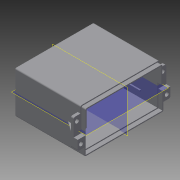
# Autodesk Inventor part: sensor2_2t
Saved by Autodesk Inventor 2015 (Build 190159000, 159)
## iProperties
Created: 2015-12-14
Part Number: sensor2_2t
Material: Generic
Document SubType Name: Modeling
Designer: mca20
Density: 1 g/cm^3
Appearance: Default
Author: mca20
Autodesk Inventor part; units mm, degrees
ref_plane "YZ Plane" through (0, 0, 0) normal (1, 0, 0) x (0, 1, 0)
ref_plane "XZ Plane" through (0, 0, 0) normal (0, 1, 0) x (-1, 0, 0)
ref_plane "XY Plane" through (0, 0, 0) normal (0, 0, 1) x (1, 0, 0)
sketch "Sketch1" plane through (0, 0, 0) normal (0, 1, 0) x (-1, 0, 0)
  line L0 (0, 0) -> (-48.5, 0)
  line L1 (-48.5, 0) -> (-48.5, -55)
  line L2 (-48.5, -55) -> (0, -55)
  line L3 (0, -55) -> (0, 0)
  line L4 (1.5, 1.5) -> (-50, 1.5)
  line L5 (-50, 1.5) -> (-50, -56.5)
  line L6 (-50, -56.5) -> (1.5, -56.5)
  line L7 (1.5, -56.5) -> (1.5, 1.5)
  dimension "d0" = 55
  dimension "d1" = 48.5
  dimension "d2" = 51.5
  dimension "d3" = 58
  dimension "d4" = 1.5
  dimension "d5" = 1.5
  constraints: 16 end point, 4 parallel, 2 horizontal, 2 perpendicular
  measures "d0" distance between parallel lines of L2 L0
  measures "d1" distance between parallel lines of L1 L3
  measures "d2" distance between parallel lines of L5 L7
  measures "d3" distance between parallel lines of L6 L4
  measures "d4" distance between parallel lines of L5 L1
  measures "d5" distance between parallel lines of L6 L2
extrude "Extrusion1" add sketch "Sketch1" against normal blind 1.5 contours L3 L2 L1 L0 | L7 L6 L5 L4
sketch "Sketch2" plane through (0, 0, 0) normal (0, 1, 0) x (1, 0, 0)
  line L0 (-1.5, -1.5) -> (50, -1.5)
  line L1 (50, 56.5) -> (-1.5, 56.5)
  line L2 (-1.5, 56.5) -> (-1.5, -1.5)
  line L3 (0, 0) -> (50, 0)
  line L4 (50, 55) -> (0, 55)
  line L5 (0, 55) -> (0, 0)
  line L6 (50, 0) -> (50, -1.5)
  line L7 (50, 56.5) -> (50, -1.5) projected
  line L8 (50, 55) -> (50, 56.5)
  line L9 (-1.5, 56.5) -> (50, 56.5) projected
  dimension "d8" = 55
  constraints: 16 end point, 2 horizontal, 2 parallel, 1 collinear, 1 perpendicular
  measures "d8" distance between parallel lines of L4 L3
extrude "Extrusion2" add sketch "Sketch2" along normal blind 28 contours L2 L1 L7 L4 L5 L3 L6 L0
sketch "Sketch3" plane through (0, 28, 0) normal (0, 1, 0) x (1, 0, 0)
  line L0 (-1.5, 56.5) -> (50, 56.5)
  line L1 (50, 56.5) -> (50, -1.5)
  line L2 (50, -1.5) -> (-1.5, -1.5)
  line L3 (-1.5, -1.5) -> (-1.5, 56.5)
  point P0 (0, 0)
  constraints: 8 end point, 2 parallel, 1 horizontal, 1 perpendicular
extrude "Extrusion3" add sketch "Sketch3" along normal blind 1.5
fillet "Fillet1" radius 1 8 edges at (24.25, 29.5, 1.5) (24.25, 29.5, -56.5) (-1.5, 29.5, -27.5) (-1.5, 14, 1.5) (24.25, -1.5, 1.5) (-1.5, -1.5, -27.5) (24.25, -1.5, -56.5) (-1.5, 14, -56.5)
sketch "Sketch4" plane through (0, 0, 0) normal (1, 0, 0) x (0, 0, -1)
  line L0 (15, 0) -> (25, 0)
  line L1 (25, 0) -> (25, 3.3)
  line L2 (25, 3.3) -> (15, 3.3)
  line L3 (15, 3.3) -> (15, 0)
  line L4 (0, 0) -> (0, 28) projected
  dimension "d14" = 3.3
  dimension "d15" = 10
  dimension "d16" = 15
  constraints: 8 end point, 2 parallel, 1 horizontal, 1 perpendicular
  measures "d14" distance between parallel lines of L2 L0
  measures "d15" distance between parallel lines of L1 L3
  measures "d16" distance between parallel lines of L4 L3
extrude "Extrusion4" add sketch "Sketch4" along normal blind 9
ref_plane "Work Plane1" through (50, 0, -27.5) normal (0, 0, -1) x (-1, 0, 0)
sketch "Sketch5" plane through (50, 0, 0) normal (0, 0, -1) x (-1, 0, 0)
  line L0 (15, 5.5) -> (35, 5.5)
  line L1 (35, 5.5) -> (35, 4.5)
  line L2 (35, 4.5) -> (15, 4.5)
  line L3 (15, 4.5) -> (15, 5.5)
  line L4 (50, 0) -> (0, 0) projected
  line L5 (50, 0) -> (50, 28) projected
  line L6 (0, 0) -> (0, 28) projected
  dimension "d20" = 1
  dimension "d21" = 4.5
  dimension "d22" = 15
  dimension "d23" = 15
  dimension "d90" = 20
  constraints: 8 end point, 2 parallel, 1 horizontal, 1 perpendicular
  measures "d20" distance between parallel lines of L2 L0
  measures "d21" distance between parallel lines of L4 L2
  measures "d22" distance between parallel lines of L5 L1
  measures "d23" distance between parallel lines of L6 L3
  measures "d90" distance between parallel lines of L1 L3
extrude "Extrusion5" add sketch "Sketch5" along normal blind 1
mirror "Mirror1" about plane through (50, 0, -27.5) normal (0, 0, -1) of "Extrusion5"
sketch "Sketch6" plane through (0, 0, -55) normal (1, 0, 0) x (0, 0, -1)
  line L0 (-24, 1) -> (-8, 1)
  line L1 (-8, 1) -> (-8, 18)
  line L2 (-8, 18) -> (-24, 18)
  line L3 (-24, 18) -> (-24, 1)
  line L4 (0, 0) -> (-30, 0) projected
  line L5 (0, 0) -> (0, 28) projected
  point P0 (-55, 0)
  dimension "d26" = 1
  dimension "d27" = 24
  dimension "d28" = 8
  dimension "d29" = 17
  constraints: 8 end point, 2 parallel, 1 horizontal, 1 perpendicular
  measures "d26" distance between parallel lines of L4 L0
  measures "d27" distance between parallel lines of L5 L3
  measures "d28" distance between parallel lines of L5 L1
  measures "d29" distance between parallel lines of L0 L2
extrude "Extrusion6" cut sketch "Sketch6" against normal blind 2
fillet "Fillet2" radius 0.5 4 edges at (-0.75, 1, -31) (-0.75, 18, -31) (-0.75, 18, -47) (-0.75, 1, -47)
sketch "Sketch7" plane through (50, -0.5, 1.5) normal (1, 0, 0) x (0, 0, -1)
  line L0 (0, 0) -> (0, 29) projected
  line L1 (0, 12.25) -> (58, 12.25)
  line L2 (58, 12.25) -> (58, 30)
  line L3 (58, 30) -> (0, 30)
  line L4 (0, 30) -> (0, 12.25)
  line L5 (0.75, 29.25) -> (57.25, 29.25)
  line L6 (57.25, 29.25) -> (57.25, 12.25)
  line L7 (57.25, 12.25) -> (0.75, 12.25)
  line L8 (0.75, 12.25) -> (0.75, 29.25)
  line L9 (58, 0) -> (58, 29) projected
  line L10 (56.5, 0.5) -> (56.5, 28.5) projected
  line L11 (1.5, 28.5) -> (56.5, 28.5)
  line L12 (56.5, 28.5) -> (56.5, 12.25)
  line L13 (56.5, 12.25) -> (1.5, 12.25)
  line L14 (1.5, 12.25) -> (1.5, 28.5)
  line L15 (1, 30) -> (57, 30) projected
  point P0 (1.5, 0.5)
  dimension "d33" = 0.75
  dimension "d34" = 0.75
  dimension "d35" = 0
  dimension "d36" = 0.75
  dimension "d37" = 0
  dimension "d38" = 0.75
  dimension "d39" = 0.75
  dimension "d40" = 17
  dimension "d41" = 0
  constraints: 24 end point, 6 parallel, 3 horizontal, 3 perpendicular, 3 point on line
  measures "d33" distance between parallel lines of L0 L8
  measures "d34" distance between parallel lines of L2 L6
  measures "d35" distance between parallel lines of L9 L2
  measures "d36" distance between parallel lines of L5 L3
  measures "d37" distance between parallel lines of L1 L7
  measures "d38" distance between parallel lines of L11 L5
  measures "d39" distance between parallel lines of L8 L14
  measures "d40" distance between parallel lines of L1 L5
  measures "d41" distance between parallel lines of L15 L3
extrude "Extrusion7" cut sketch "Sketch7" against normal blind 3 contours L0 L4 L3 L2 L1 L6 L5 L8
fillet "Fillet3" radius 1 2 edges at (48.5, 28.75, -55.75) (48.5, 28.75, 0.75)
sketch "Sketch8" plane through (50, -1.5, 0.5) normal (1, 0, 0) x (0, 0, -1)
  line L0 (57.0002, 17.5) -> (-0.9998, 17.5)
  line L1 (-0.9998, 17.5) -> (-0.9998, 0.75)
  line L2 (-0.9998, 0.75) -> (57.0002, 0.75)
  line L3 (57.0002, 0.75) -> (57.0002, 17.5)
  line L4 (56, 0) -> (0, 0) projected
  line L5 (-0.2498, 17.5) -> (56.2502, 17.5)
  line L6 (56.2502, 17.5) -> (56.2502, 0.75)
  line L7 (56.2502, 0.75) -> (-0.2498, 0.75)
  line L8 (-0.2498, 0.75) -> (-0.2498, 17.5)
  line L9 (0.5, 17.5) -> (55.5, 17.5)
  line L10 (55.5, 17.5) -> (55.5, 1.5)
  line L11 (55.5, 1.5) -> (0.5, 1.5)
  line L12 (0.5, 1.5) -> (0.5, 17.5)
  dimension "d45" = 58
  dimension "d46" = 16.75
  dimension "d47" = 0.75
  dimension "d48" = 0
  dimension "d49" = 0.75
  dimension "d50" = 0.75
  constraints: 24 end point, 6 parallel, 3 horizontal, 3 perpendicular, 2 point on line
  measures "d45" distance between parallel lines of L3 L1
  measures "d46" distance between parallel lines of L2 L0
  measures "d47" distance between parallel lines of L4 L2
  measures "d48" distance between parallel lines of L0 L5
  measures "d49" distance between parallel lines of L1 L8
  measures "d50" distance between parallel lines of L3 L6
extrude "Extrusion8" cut sketch "Sketch8" against normal blind 3 contours L6 L2 L8 L0 L12 L11 L10
sketch "Sketch9" plane through (50, -0.5, -56.5) normal (0, 0, -1) x (-1, 0, 0)
  line L0 (3, 12.25) -> (5, 12.25)
  line L1 (5, 12.25) -> (5, 25)
  line L2 (5, 25) -> (3, 25)
  line L3 (3, 25) -> (3, 12.25)
  line L4 (5, 12.25) -> (0, 12.25)
  line L5 (0, 12.25) -> (0, 5)
  line L6 (0, 5) -> (5, 5)
  line L7 (5, 5) -> (5, 12.25)
  line L8 (0, 0) -> (0, 12.25) projected
  point P0 (50, 0.5)
  point P1 (3, 30)
  point P2 (0, -1)
  dimension "d60" = 2
  dimension "d61" = 12.75
  dimension "d62" = 5
  dimension "d63" = 5
  dimension "d64" = 7.25
  dimension "d65" = 0
  constraints: 16 end point, 4 parallel, 2 horizontal, 2 perpendicular
  measures "d60" distance of L2.end L1.end
  measures "d61" distance of L1.end L0.end
  measures "d62" distance from line of L2 point (3, 30)
  measures "d63" distance between parallel lines of L7 L5
  measures "d64" distance between parallel lines of L6 L4
  measures "d65" distance between parallel lines of L8 L5
extrude "Extrusion9" add sketch "Sketch9" along normal blind 5
fillet "Fillet4" radius 1 2 edges at (46, 24.5, -61.5) (47.5, 4.5, -61.5)
sketch "Sketch10" plane through (47, -0.5, 1.5) normal (1, 0, 0) x (0, 0, -1)
  circle A0 centre (60.5, 21.5) radius 1.5
  line L0 (63, 24) -> (63, 12.25) projected
  line L1 (58, 25) -> (62, 25) projected
  point P0 (1.5, 0.5)
  dimension "d69" = 3
  dimension "d70" = 2.5
  dimension "d71" = 3.5
  constraints: 1 centre point
  measures "d69" diameter of A0
  measures "d70" distance from line of L0 A0.centre
  measures "d71" distance from line of L1 A0.centre
extrude "Extrusion10" cut sketch "Sketch10" against normal blind 2
sketch "Sketch11" plane through (50, -1.5, 0.5) normal (1, 0, 0) x (0, 0, -1)
  circle A0 centre (59.5, 9.5) radius 1.5
  line L0 (57, 6) -> (61, 6) projected
  line L1 (62, 13.25) -> (62, 7) projected
  point P0 (0.5, 1.5)
  dimension "d74" = 3
  dimension "d75" = 3.5
  dimension "d76" = 2.5
  constraints: 1 centre point
  measures "d74" diameter of A0
  measures "d75" distance from line of L0 A0.centre
  measures "d76" distance from line of L1 A0.centre
extrude "Extrusion11" cut sketch "Sketch11" against normal blind 5
mirror "Mirror2" about plane through (50, 0, -27.5) normal (0, 0, -1) of "Extrusion9", "Extrusion11", "Fillet4", "Extrusion10"
ref_plane "Work Plane2" through (0, 14, 0) normal (0, -1, 0) x (1, 0, 0)
sketch "Sketch12" plane through (0, 14, 0) normal (0, -1, 0) x (1, 0, 0)
  line L0 (45, -61.5) -> (39.2874, -57.5)
  line L1 (45, -61.5) -> (51.9738, -61.5) construction
  point P0 (0, 0)
  dimension "d80" = 145
  constraints: 4 end point, 1 equal length, 1 horizontal
  measures "d80" angle of L1 L0
extrude "Rib1" add sketch "Sketch12" along normal mid plane 2 rib yes fills toward (42.1724, -59.459) open curves L0
mirror "Mirror3" about plane through (50, 0, -27.5) normal (0, 0, -1) of "Rib1"
ref_plane "Work Plane6" through (15, 5, 0) normal (0, 1, 0) x (1, 0, 0)
sketch "Sketch15" plane through (15, 5, 0) normal (0, 1, 0) x (1, 0, 0)
  line L0 (0, 1) -> (-0.7071, 0.2929)
  line L1 (0, 1) -> (1, 1) construction
  point P0 (-15, 0)
  dimension "d100" = 1
  dimension "d101" = 135
  constraints: 4 end point, 1 equal length, 1 horizontal
  measures "d100" distance of L0.start L0.end
  measures "d101" angle of L0 L1
extrude "Rib3" add sketch "Sketch15" along normal mid plane 1 rib yes fills toward (-0.3182, 0.6111) open curves L0
mirror "Mirror5" about plane through (50, 0, -27.5) normal (0, 0, -1) of "Rib3"
equation "\"d34\" = d33"
equation "\"d36\" = d33"
equation "\"d38\" = d36"
equation "\"d39\" = d33"
body "Solid1"
